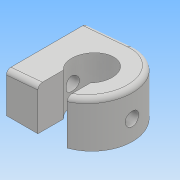
# Autodesk Inventor part: Hand - Digit 4
Saved by Autodesk Inventor 2017 (Build 210142000, 142)
## iProperties
Created: 2016-09-27
Part Number: Hand - Digit 4
Material: Generic
Document SubType Name: Modeling
Designer: cmcdona
Density: 1 g/cm^3
Appearance: Default
Author: cmcdona
Autodesk Inventor part; units mm, degrees
ref_plane "YZ Plane" through (0, 0, 0) normal (1, 0, 0) x (0, 1, 0)
ref_plane "XZ Plane" through (0, 0, 0) normal (0, 1, 0) x (-1, 0, 0)
ref_plane "XY Plane" through (0, 0, 0) normal (0, 0, 1) x (1, 0, 0)
sketch "Sketch1" plane through (0, 0, 0) normal (0, 0, 1) x (1, 0, 0)
  line L0 (0, 0) -> (114, 0)
  arc A0 (114, 0) -> (114, 18) centre (114, 9) ccw
  arc A1 (0, 21) -> (0, 0) centre (0, 10.5) ccw
  line L1 (0, 21) -> (20.7846, 18)
  line L2 (20.7846, 18) -> (114, 18)
  circle A2 centre (114, 9) radius 4.5
  dimension "d0" = 114
  dimension "d1" = 18
  dimension "d2" = 9
  dimension "d3" = 21
  dimension "d4" = 10.5
  dimension "d5" = 21
  dimension "d6" = 9
  constraints: 6 end point, 4 point on circle, 3 centre point, 2 horizontal, 1 coincident
  measures "d0" distance of L0.start L0.end
  measures "d1" distance of L0.end L2.end
  measures "d2" radius of A0
  measures "d3" distance of L0.start L1.start
  measures "d4" radius of A1
  measures "d5" distance of L1.start L1.end
  measures "d6" diameter of A2
extrude "Extrusion1" add sketch "Sketch1" against normal blind 12
sketch "Sketch2" plane through (0, 0, 0) normal (0, 0, 1) x (1, 0, 0)
  line L0 (111, 0) -> (117, 0)
  line L1 (117, 0) -> (117, 6)
  line L2 (117, 6) -> (111, 6)
  line L3 (111, 6) -> (111, 0)
  point P0 (0, 0)
  dimension "d9" = 6
  dimension "d10" = 6
  constraints: 8 end point, 2 parallel, 1 horizontal, 1 perpendicular
  measures "d9" distance of L2.end L1.end
  measures "d10" distance of L1.end L0.end
extrude "Extrusion2" cut sketch "Sketch2" against normal through all
sketch "Sketch3" plane through (0, 0, -12) normal (0, -1, 0) x (1, 0, 0)
  line L0 (-10.5, 12) -> (-10.5, 4)
  line L1 (-10.5, 12) -> (-10.5, 0) projected
  line L2 (-10.5, 4) -> (49, 4)
  line L3 (49, 4) -> (140.4404, 12)
  line L4 (140.4404, 12) -> (-10.5, 12)
  point P0 (0, 12)
  dimension "d13" = 8
  dimension "d14" = 59.5
  dimension "d15" = 175
  constraints: 8 end point, 1 parallel, 1 perpendicular, 1 point on line
  measures "d13" distance of L0.start L0.end
  measures "d14" distance of L0.end L2.end
  measures "d15" angle of L3 L2
extrude "Extrusion3" cut sketch "Sketch3" against normal through all
sketch "Sketch4" plane through (0, 0, -12) normal (0, 0, -1) x (-1, 0, 0)
  line L0 (10.5, 0) -> (-104, 0)
  line L1 (-104, 0) -> (-104, 21)
  line L2 (-104, 21) -> (10.5, 21)
  line L3 (10.5, 21) -> (10.5, 0)
  point P0 (0, 0)
  dimension "d18" = 114.5
  dimension "d19" = 21
  constraints: 8 end point, 2 parallel, 1 horizontal, 1 perpendicular
  measures "d18" distance of L1.end L2.end
  measures "d19" distance of L0.end L1.end
extrude "Extrusion4" cut sketch "Sketch4" against normal through all
sketch "Sketch5" plane through (104, 0, -12) normal (-1, 0, 0) x (0, 0, 1)
  circle A0 centre (4.4, 9) radius 1.5
  point P0 (12, 0)
  dimension "d29" = 3
  constraints: 1 centre point
  measures "d29" diameter of A0
extrude "Extrusion5" cut sketch "Sketch5" against normal through all
fillet "Fillet1" radius 1 3 edges at (109, 18, -2.7507) (122.8704, 10.5219, -1.5372) (107.5, 0, -2.8819)
sketch "Sketch6" plane through (104, 18, -12) normal (0, 1, 0) x (1, 0, 0)
  circle A0 centre (5, -4) radius 1.5
  point P0 (-104, -12)
  dimension "d26" = 3
  constraints: 1 centre point
  measures "d26" diameter of A0
extrude "Extrusion6" cut sketch "Sketch6" against normal blind 5
body "Solid1"
